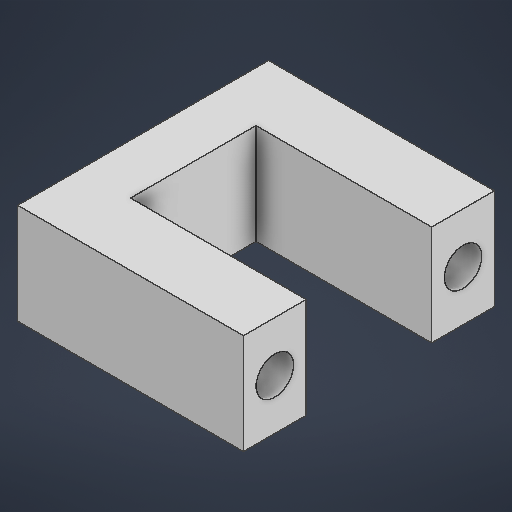
# Autodesk Inventor part: servo_support_4
Saved by Autodesk Inventor 2026.1 (Build 301233000, 233)
## iProperties
Created: 2025-10-11
Part Number: servo_support_4
Material: Generic
Document SubType Name: Modeling
Designer: emanuel
Density: 1 g/cm^3
Appearance: Default
Author: emanuel
Autodesk Inventor part; units mm, degrees
ref_plane "YZ Plane" through (0, 0, 0) normal (1, 0, 0) x (0, 1, 0)
ref_plane "XZ Plane" through (0, 0, 0) normal (0, 1, 0) x (-1, 0, 0)
ref_plane "XY Plane" through (0, 0, 0) normal (0, 0, 1) x (1, 0, 0)
sketch "Sketch1" plane through (0, 0, 0) normal (0, 1, 0) x (-1, 0, 0)
  line L0 (0, 0) -> (18, 0)
  line L1 (18, 0) -> (18, -20)
  line L2 (18, -20) -> (0, -20)
  line L3 (0, -20) -> (0, 0)
  line L4 (0, 0) -> (0, -5)
  line L5 (0, -5) -> (14, -5)
  line L6 (14, -5) -> (14, -15)
  line L7 (14, -15) -> (0, -15)
  line L8 (0, -15) -> (0, -5)
  dimension "d0" = 18
  dimension "d1" = 20
  dimension "d2" = 5
  dimension "d3" = 14
  dimension "d4" = 10
  constraints: 18 end point, 4 parallel, 2 horizontal, 2 perpendicular, 1 point on line
  measures "d0" distance of L1.end L2.end
  measures "d1" distance of L0.end L1.end
  measures "d2" distance of L0.start L4.end
  measures "d3" distance of L6.end L7.end
  measures "d4" distance of L5.end L6.end
extrude "Extrusion1" add sketch "Sketch1" along normal blind 8 contours L0 L1 L2 L3 L7 L6 L5
sketch "Sketch2" plane through (0, 0, 0) normal (1, 0, 0) x (0, 0, -1)
  line L0 (20, 8) -> (0, 8) projected
  line L1 (0, 8) -> (2.5, 8)
  line L2 (2.5, 8) -> (2.5, 4)
  line L3 (2.5, 4) -> (0, 4)
  line L4 (0, 4) -> (0, 8)
  line L5 (20, 0) -> (20, 8) projected
  line L6 (20, 8) -> (17.5, 8)
  line L7 (17.5, 8) -> (17.5, 4)
  line L8 (17.5, 4) -> (20, 4)
  line L9 (20, 4) -> (20, 8)
  circle A0 centre (2.5, 4) radius 1.5
  circle A1 centre (17.5, 4) radius 1.5
  point P0 (0, 0)
  dimension "d7" = 2.5
  dimension "d8" = 4
  dimension "d9" = 2.5
  dimension "d10" = 4
  dimension "d11" = 3
  dimension "d12" = 3
  constraints: 16 end point, 4 parallel, 2 centre point, 2 coincident, 2 horizontal, 2 perpendicular
  measures "d7" distance of L2.end L3.end
  measures "d8" distance of L1.end L2.end
  measures "d9" distance of L8.end L7.end
  measures "d10" distance of L7.end L6.end
  measures "d11" diameter of A0
  measures "d12" diameter of A1
extrude "Extrusion2" cut sketch "Sketch2" against normal blind 14 contours A1 L8 L7 | L7 L8 A1 | A0 L3 L2 | L2 L3 A0
body "Solid1"
